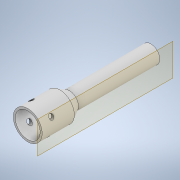
# Autodesk Inventor part: oxidizer
Saved by Autodesk Inventor 2021 (Build 250183000, 183)
## iProperties
Created: 2023-07-01
Part Number: oxidizer
Material: Generic
Document SubType Name: Modeling
Designer: harsh
Density: 1 g/cm^3
Appearance: Default
Author: harsh
Autodesk Inventor part; units mm, degrees
ref_plane "XZ Plane" through (0, 0, 0) normal (0, 1, 0) x (-1, 0, 0)
ref_plane "XY Plane" through (0, 0, 0) normal (0, 0, 1) x (1, 0, 0)
sketch "Sketch1" plane through (0, 0, 0) normal (1, 0, 0) x (0, 1, 0)
  line L0 (5.5, 0) -> (5.5, -14)
  line L1 (3, -18.3301) -> (3, -54.5301)
  line L2 (5.5, -14) -> (3, -18.3301)
  line L3 (6.4, -14.2412) -> (6.4, 0)
  line L4 (3.9, -54.5301) -> (3.9, -18.5713)
  line L5 (3.9, -18.5713) -> (6.4, -14.2412)
  line L6 (5.5, 0) -> (6.4, 0)
  line L7 (3, -54.5301) -> (3.9, -54.5301)
  line L8 (0, 0) -> (0, -13.4329) construction
  dimension "d7" = 5.5
  dimension "d8" = 3
  dimension "d9" = 150
  dimension "d10" = 0.9
  dimension "d11" = 0.9
  dimension "d12" = 0.9
  dimension "d13" = 14
  dimension "d14" = 36.2
  constraints: 18 end point, 1 horizontal, 1 perpendicular, 1 vertical
  measures "d7" distance between parallel lines of L0 L8
  measures "d8" distance between parallel lines of L1 L8
  measures "d9" angle of L2 L0
  measures "d10" distance between parallel lines of L0 L3
  measures "d11" distance between parallel lines of L5 L2
  measures "d12" distance between parallel lines of L4 L1
  measures "d13" distance of L0.start L0.end
  measures "d14" distance of L1.start L1.end
revolve "Revolution1" add sketch "Sketch1" angle 360 about axis through (0, 0, 0) along (0, 0, -1)
ref_plane "Work Plane2" through (7, 0, 0) normal (1, 0, 0) x (0, 1, 0)
sketch "Sketch2" plane through (7, 0, 0) normal (1, 0, 0) x (0, 1, 0)
  line L0 (0, 0) -> (0, -5) construction
  line L1 (0, -5) -> (3.4, -5) construction
  circle A0 centre (3.4, -5) radius 1
  dimension "d18" = 5
  dimension "d19" = 3.4
  dimension "d20" = 2
  constraints: 4 end point, 1 centre point, 1 coincident, 1 perpendicular, 1 vertical
  measures "d18" distance of L0.start L0.end
  measures "d19" distance of L0.end L1.end
  measures "d20" diameter of A0
extrude "Extrusion1" cut sketch "Sketch2" against normal blind 5
pattern_circular "Circular Pattern1" count 4 over 360 about axis through (0, 0, -7) along (0, 0, -1) of "Extrusion1"
body "Solid1"
